Autodesk Inventor part; units mm, degrees
(part 2 of 18)
  ellipse E96 centre (-10059.4953, -10011.6684) end of major axis (-10059.5216, -10011.169) minor radius 0.0016 (-10059.5115, -10011.3383) -> (-10059.5141, -10011.3335) ccw
  line L123 (-10061.6074, -10010.6749) -> (-10061.6853, -10010.6709)
  line L124 (-10061.783, -10009.7539) -> (-10061.5792, -10009.7642)
  line L125 (-10061.6156, -10010.9399) -> (-10061.5672, -10009.3749)
  ellipse E97 centre (-10061.4209, -10009.295) end of major axis (-10061.3805, -10008.496) minor radius 0.143 (-10061.3805, -10008.496) -> (-10061.5409, -10009.0123) ccw
  line L126 (-10061.571, -10010.9422) -> (-10061.6156, -10010.9399)
  ellipse E98 centre (-10059.4556, -10009.3943) end of major axis (-10059.4152, -10008.5953) minor radius 0.143 (-10059.3426, -10008.7344) -> (-10059.5711, -10009.0745) ccw
  line L127 (-10059.4152, -10008.5953) -> (-10061.3805, -10008.496)
  line L128 (-10061.571, -10009.4991) -> (-10061.8166, -10009.4867)
  line L129 (-10061.6156, -10010.9399) -> (-10061.8118, -10010.93)
  line L130 (-10063.3919, -10010.8501) -> (-10063.6427, -10010.8374)
  ellipse E99 centre (-10075.0796, -10008.6044) end of major axis (-10074.9741, -10006.5171) minor radius 0.3735 (-10074.9741, -10006.5171) -> (-10075.403, -10007.9525) ccw
  ellipse E100 centre (-10074.1952, -10008.6491) end of major axis (-10074.0897, -10006.5618) minor radius 0.3735 (-10073.8946, -10006.9512) -> (-10074.5173, -10007.9854) ccw
  line L131 (-10074.9741, -10006.5171) -> (-10074.0897, -10006.5618)
  ellipse E101 centre (-10074.1952, -10008.6491) end of major axis (-10074.1195, -10007.151) minor radius 0.2681 (-10074.0146, -10007.2936) -> (-10074.4107, -10009.8693) ccw
  ellipse E102 centre (-10059.4556, -10009.3943) end of major axis (-10059.4303, -10008.895) minor radius 0.0894 (-10059.3634, -10009.2087) -> (-10059.5442, -10009.3788) ccw
  line L132 (-10059.8989, -10015.0944) -> (-10059.8016, -10014.6093)
  line L133 (-10059.8016, -10014.6093) -> (-10059.814, -10014.6001)
  ellipse E103 centre (-10059.3774, -10016.4493) end of major axis (-10059.1723, -10015.676) minor radius 0.1421 (-10059.1558, -10016.0937) -> (-10059.1723, -10015.676) ccw
  line L134 (-10059.1723, -10015.676) -> (-10059.8752, -10015.4896)
  line L135 (-10062.35, -10019.5456) -> (-10062.8067, -10019.5173)
  line L136 (-10060.3914, -10027.4914) -> (-10060.3323, -10027.2827)
  ellipse E104 centre (-10060.3058, -10027.7257) end of major axis (-10060.5274, -10028.4943) minor radius 0.1461 (-10060.3074, -10027.284) -> (-10060.3936, -10027.516) ccw
  ellipse E105 centre (-10059.3611, -10027.9981) end of major axis (-10059.2226, -10027.5176) minor radius 0.0913 (-10059.2273, -10027.8389) -> (-10059.4494, -10027.9748) ccw
  ellipse E106 centre (-10059.3611, -10027.9981) end of major axis (-10059.1395, -10027.2294) minor radius 0.1461 (-10059.1442, -10027.7299) -> (-10059.4076, -10027.6709) ccw
  line L137 (-10059.1395, -10027.2294) -> (-10059.5247, -10027.1183)
  ellipse E107 centre (-10061.1947, -10025.0322) end of major axis (-10061.4841, -10025.778) minor radius 0.0025 (-10061.4641, -10025.7239) -> (-10061.4841, -10025.778) ccw
  ellipse E108 centre (-10061.1947, -10025.0322) end of major axis (-10060.9052, -10024.2864) minor radius 0.0025 (-10061.4579, -10025.7077) -> (-10061.4588, -10025.71) ccw
  line L138 (-10060.6601, -10023.6469) -> (-10060.6559, -10023.6361)
  line L139 (-10060.6559, -10023.6361) -> (-10059.7237, -10023.9979)
  ellipse E109 centre (-10059.3301, -10025.7558) end of major axis (-10059.0407, -10025.01) minor radius 0.0025 (-10059.215, -10025.4653) -> (-10059.2158, -10025.4549) ccw
  line L140 (-10061.4747, -10025.7816) -> (-10061.4841, -10025.778)
  line L141 (-10059.0407, -10025.01) -> (-10059.9651, -10024.6512)
  line L142 (-10060.6559, -10023.6361) -> (-10060.6965, -10023.6203)
  line L143 (-10060.8833, -10023.5478) -> (-10065.815, -10021.6339)
  ellipse E110 centre (-10059.9849, -10023.8481) end of major axis (-10060.3776, -10022.9558) minor radius 0.1687 (-10059.9009, -10023.6263) -> (-10060.3456, -10022.9572) ccw
  line L144 (-10060.3456, -10022.9572) -> (-10064.6064, -10021.3037)
  line L145 (-10059.9009, -10023.6263) -> (-10059.7237, -10023.9979)
  line L146 (-10059.7237, -10023.9979) -> (-10059.9563, -10024.6128)
  line L147 (-10059.948, -10024.5763) -> (-10059.7237, -10023.9979)
  ellipse E111 centre (-10059.3301, -10025.7558) end of major axis (-10059.1492, -10025.2896) minor radius 0.0015 (-10059.2152, -10025.4628) -> (-10059.2156, -10025.4573) ccw
  line L148 (-10061.1673, -10013.709) -> (-10061.4116, -10012.4308)
  ellipse E112 centre (-10061.4191, -10012.3797) end of major axis (-10061.5691, -10011.5939) minor radius 0.0022 (-10061.4497, -10012.231) -> (-10061.4116, -10012.4308) ccw
  ellipse E113 centre (-10061.4191, -10012.3797) end of major axis (-10061.5691, -10011.5939) minor radius 0.0022 (-10061.5691, -10011.5939) -> (-10061.4792, -10012.076) ccw
  line L149 (-10061.5626, -10011.5927) -> (-10061.5691, -10011.5939)
  line L150 (-10061.4353, -10010.9692) -> (-10061.5403, -10010.0292)
  ellipse E114 centre (-10074.1883, -10011.2004) end of major axis (-10074.3345, -10009.7075) minor radius 0.2416 (-10074.3956, -10009.773) -> (-10074.4256, -10009.8711) ccw
  ellipse E115 centre (-10074.1883, -10011.2004) end of major axis (-10074.392, -10009.1204) minor radius 0.3366 (-10074.4689, -10009.1938) -> (-10074.4718, -10009.1998) ccw
  ellipse E116 centre (-10059.4546, -10009.7574) end of major axis (-10059.4058, -10010.255) minor radius 0.0805 (-10059.453, -10010.1908) -> (-10059.4275, -10010.2411) ccw
  ellipse E117 centre (-10059.4546, -10009.7574) end of major axis (-10059.5033, -10009.2598) minor radius 0.0805 (-10059.5175, -10009.2701) -> (-10059.5437, -10009.3842) ccw
  ellipse E118 centre (-10061.3909, -10025.8081) end of major axis (-10061.2388, -10025.0226) minor radius 0.0868 (-10061.4894, -10025.8618) -> (-10061.5648, -10026.4557) ccw
  line L151 (-10061.4894, -10025.8618) -> (-10061.4567, -10025.6836)
  line L152 (-10061.2304, -10013.1017) -> (-10061.302, -10012.8602)
  ellipse E119 centre (-10061.3135, -10012.8141) end of major axis (-10061.5409, -10012.0472) minor radius 0.0022 (-10061.3592, -10012.6675) -> (-10061.302, -10012.8602) ccw
  ellipse E120 centre (-10061.3135, -10012.8141) end of major axis (-10061.5409, -10012.0472) minor radius 0.0022 (-10061.3802, -10012.5962) -> (-10061.3795, -10012.5988) ccw
  ellipse E121 centre (-10061.3135, -10012.8141) end of major axis (-10061.5409, -10012.0472) minor radius 0.0022 (-10061.5409, -10012.0477) -> (-10061.4673, -10012.3011) ccw
  line L153 (-10059.8961, -10014.0829) -> (-10060.2291, -10014.1817)
  line L154 (-10067.4297, -10016.1096) -> (-10067.4268, -10016.1197)
  line L155 (-10064.2229, -10015.3662) -> (-10067.0815, -10016.2141)
  line L156 (-10059.8993, -10014.0717) -> (-10059.8961, -10014.0829)
  line L157 (-10059.8961, -10014.0829) -> (-10059.936, -10014.1466)
  line L158 (-10059.8961, -10014.0829) -> (-10059.9646, -10013.8519)
  line L159 (-10061.4597, -10010.5107) -> (-10061.4635, -10010.4932)
  ellipse E122 centre (-10061.3479, -10010.4186) end of major axis (-10061.5106, -10009.6353) minor radius 0.1285 (-10061.5089, -10010.2574) -> (-10061.4635, -10010.4932) ccw
  line L160 (-10060.3618, -10010.9128) -> (-10060.3756, -10010.8496)
  ellipse E123 centre (-10059.4151, -10010.0173) end of major axis (-10059.3135, -10010.5069) minor radius 0.0803 (-10059.4497, -10010.2168) -> (-10059.2869, -10010.3723) ccw
  ellipse E124 centre (-10061.4428, -10028.7052) end of major axis (-10061.4376, -10029.5052) minor radius 0.1258 (-10061.5687, -10028.685) -> (-10061.4376, -10029.5052) ccw
  line L161 (-10061.5687, -10028.685) -> (-10061.5705, -10027.9704)
  line L162 (-10061.5725, -10027.1323) -> (-10061.5726, -10027.1107)
  line L163 (-10061.5726, -10027.1107) -> (-10061.5433, -10027.1105)
  ellipse E125 centre (-10059.4677, -10028.6922) end of major axis (-10059.4625, -10029.4922) minor radius 0.1258 (-10059.5871, -10028.4073) -> (-10059.5936, -10028.672) ccw
  line L164 (-10061.5726, -10027.1107) -> (-10062.1103, -10027.1142)
  line L165 (-10063.1147, -10027.1209) -> (-10063.6302, -10027.1243)
  ellipse E126 centre (-10075.1696, -10028.7957) end of major axis (-10075.1558, -10030.8856) minor radius 0.3286 (-10075.4962, -10028.958) -> (-10075.432, -10029.9867) ccw
  ellipse E127 centre (-10074.2808, -10028.7898) end of major axis (-10074.267, -10030.8798) minor radius 0.3286 (-10074.6056, -10029.0344) -> (-10074.5441, -10029.973) ccw
  ellipse E128 centre (-10074.2808, -10028.7898) end of major axis (-10074.2709, -10030.2898) minor radius 0.2359 (-10074.5075, -10028.3133) -> (-10074.258, -10030.2874) ccw
  ellipse E129 centre (-10059.4677, -10028.6922) end of major axis (-10059.4645, -10029.1922) minor radius 0.0786 (-10059.5435, -10028.8078) -> (-10059.4024, -10028.9872) ccw
  ellipse E130 centre (-10061.4829, -10026.279) end of major axis (-10061.5501, -10027.0761) minor radius 0.0022 (-10061.4921, -10026.3627) -> (-10061.5501, -10027.0761) ccw
  line L166 (-10061.5412, -10027.0769) -> (-10061.5501, -10027.0761)
  line L167 (-10061.1675, -10013.708) -> (-10064.1267, -10014.2572)
  line L168 (-10061.0399, -10013.9291) -> (-10061.1256, -10013.7034)
  line L169 (-10061.0399, -10013.9291) -> (-10061.3186, -10012.3815)
  ellipse E131 centre (-10061.4026, -10012.3529) end of major axis (-10061.5486, -10011.5664) minor radius 0.0775 (-10061.3186, -10012.3815) -> (-10061.5655, -10011.726) ccw
  ellipse E132 centre (-10061.4026, -10012.3529) end of major axis (-10061.2567, -10013.1395) minor radius 0.0775 (-10061.5654, -10011.7276) -> (-10061.5651, -10011.7329) ccw
  line L170 (-10061.5651, -10011.7329) -> (-10061.5627, -10011.7772)
  line L171 (-10061.006, -10013.9229) -> (-10061.0399, -10013.9291)
  line L172 (-10061.5148, -10011.5601) -> (-10061.5486, -10011.5664)
  line L173 (-10061.0399, -10013.9291) -> (-10062.4396, -10014.1889)
  line L174 (-10061.5324, -10011.3464) -> (-10062.0925, -10011.4011)
  line L175 (-10061.413, -10010.968) -> (-10061.51, -10010.0167)
  ellipse E133 centre (-10061.4701, -10009.9537) end of major axis (-10061.5479, -10009.1575) minor radius 0.046 (-10061.5593, -10009.2154) -> (-10061.51, -10010.0167) ccw
  line L176 (-10061.5682, -10011.6005) -> (-10062.0791, -10011.6504)
  ellipse E134 centre (-10075.2814, -10011.3029) end of major axis (-10075.4846, -10009.2228) minor radius 0.1201 (-10075.4962, -10009.236) -> (-10075.5025, -10009.9969) ccw
  ellipse E135 centre (-10074.3871, -10011.2156) end of major axis (-10074.5903, -10009.1355) minor radius 0.1201 (-10074.6056, -10009.1595) -> (-10074.6228, -10009.4041) ccw
  ellipse E136 centre (-10074.3871, -10011.2156) end of major axis (-10074.533, -10009.7227) minor radius 0.0862 (-10074.479, -10009.8773) -> (-10074.556, -10009.8863) ccw
  ellipse E137 centre (-10059.4829, -10009.7596) end of major axis (-10059.5315, -10009.2619) minor radius 0.0287 (-10059.5388, -10009.3031) -> (-10059.5392, -10009.3196) ccw
  line L177 (-10062.0933, -10026.8089) -> (-10061.5337, -10026.8636)
  ellipse E138 centre (-10061.4701, -10028.2403) end of major axis (-10061.5479, -10029.0365) minor radius 0.046 (-10061.5147, -10028.2236) -> (-10061.5593, -10028.9786) ccw
  line L178 (-10061.5147, -10028.2236) -> (-10061.4163, -10027.2258)
  ellipse E139 centre (-10075.2814, -10026.8911) end of major axis (-10075.4846, -10028.9712) minor radius 0.1201 (-10075.5025, -10028.1971) -> (-10075.4962, -10028.958) ccw
  ellipse E140 centre (-10074.3871, -10026.9784) end of major axis (-10074.5903, -10029.0585) minor radius 0.1201 (-10074.6228, -10028.7899) -> (-10074.6056, -10029.0344) ccw
  ellipse E141 centre (-10074.3871, -10026.9784) end of major axis (-10074.533, -10028.4713) minor radius 0.0862 (-10074.556, -10028.3077) -> (-10074.479, -10028.3167) ccw
  ellipse E142 centre (-10059.4829, -10028.4344) end of major axis (-10059.4343, -10027.9368) minor radius 0.0287 (-10059.4284, -10027.9558) -> (-10059.4497, -10027.9771) ccw
  ellipse E143 centre (-10059.4829, -10028.4344) end of major axis (-10059.5315, -10028.9321) minor radius 0.0287 (-10059.534, -10028.7144) -> (-10059.5203, -10028.9087) ccw
  line L179 (-10064.1321, -10023.9836) -> (-10061.1995, -10024.5278)
  ellipse E144 centre (-10061.4026, -10025.8411) end of major axis (-10061.5486, -10026.6276) minor radius 0.0775 (-10061.5648, -10026.4557) -> (-10061.3382, -10025.9171) ccw
  line L180 (-10061.3382, -10025.9171) -> (-10061.0521, -10024.4386)
  line L181 (-10061.5148, -10026.6339) -> (-10061.5486, -10026.6276)
  line L182 (-10061.3493, -10013.5219) -> (-10061.4817, -10011.9546)
  ellipse E145 centre (-10061.4829, -10011.915) end of major axis (-10061.5501, -10011.1179) minor radius 0.0022 (-10061.492, -10011.8329) -> (-10061.4817, -10011.9546) ccw
  ellipse E146 centre (-10061.4829, -10011.915) end of major axis (-10061.5501, -10011.1179) minor radius 0.0022 (-10061.5501, -10011.1179) -> (-10061.492, -10011.8327) ccw
  line L183 (-10061.2053, -10013.5098) -> (-10061.3493, -10013.5219)
  line L184 (-10061.5412, -10011.1171) -> (-10061.5501, -10011.1179)
  line L185 (-10061.3493, -10013.5219) -> (-10063.059, -10013.6661)
  line L186 (-10064.1551, -10013.7586) -> (-10064.1846, -10013.7611)
  line L187 (-10061.7547, -10009.9957) -> (-10061.5864, -10009.9968)
  line L188 (-10061.558, -10011.1248) -> (-10061.5686, -10009.5555)
  ellipse E147 centre (-10061.4428, -10009.4888) end of major axis (-10061.4376, -10008.6888) minor radius 0.1258 (-10061.5458, -10009.0552) -> (-10061.5686, -10009.5555) ccw
  line L189 (-10061.5498, -10011.1249) -> (-10061.558, -10011.1248)
  line L190 (-10061.558, -10011.1248) -> (-10062.1079, -10011.1212)
  line L191 (-10063.1128, -10011.1146) -> (-10063.9018, -10011.1094)
  ellipse E148 centre (-10075.1696, -10009.3983) end of major axis (-10075.1834, -10011.4883) minor radius 0.3286 (-10075.432, -10008.2073) -> (-10075.4962, -10009.236) ccw
  ellipse E149 centre (-10074.2808, -10009.4042) end of major axis (-10074.2946, -10011.4941) minor radius 0.3286 (-10074.5441, -10008.2209) -> (-10074.6056, -10009.1595) ccw
  ellipse E150 centre (-10074.2808, -10009.4042) end of major axis (-10074.2709, -10007.9042) minor radius 0.2359 (-10074.2349, -10007.9221) -> (-10074.5075, -10009.8807) ccw
  ellipse E151 centre (-10060.4553, -10009.4953) end of major axis (-10060.4606, -10010.2952) minor radius 0.1258 (-10060.5811, -10009.562) -> (-10060.5678, -10009.8834) ccw
  ellipse E152 centre (-10059.4677, -10009.5018) end of major axis (-10059.4645, -10009.0018) minor radius 0.0786 (-10059.5212, -10009.1492) -> (-10059.5435, -10009.3862) ccw
  line L192 (-10060.3705, -10027.2925) -> (-10060.3681, -10027.2809)
  ellipse E153 centre (-10059.4151, -10028.1767) end of major axis (-10059.3135, -10027.6871) minor radius 0.0803 (-10059.2869, -10027.8217) -> (-10059.4497, -10027.9772) ccw
  ellipse E154 centre (-10061.3135, -10025.3799) end of major axis (-10061.5409, -10026.1468) minor radius 0.0022 (-10061.4677, -10025.8942) -> (-10061.5409, -10026.1463) ccw
  line L193 (-10065.4273, -10022.5831) -> (-10067.279, -10022.0339)
  line L194 (-10067.4279, -10022.0746) -> (-10067.4306, -10022.084)
  ellipse E155 centre (-10063.9396, -10011.2006) end of major axis (-10064.1437, -10010.36) minor radius 0.1481 (-10064.0618, -10011.3216) -> (-10064.0429, -10011.3917) ccw
  ellipse E156 centre (-10063.9396, -10011.2006) end of major axis (-10064.1437, -10010.36) minor radius 0.1481 (-10064.1077, -10011.131) -> (-10064.0971, -10011.178) ccw
  ellipse E157 centre (-10064.7515, -10028.8711) end of major axis (-10064.763, -10028.4142) minor radius 0.0765 (-10064.8032, -10028.491) -> (-10064.8181, -10029.044) ccw
  ellipse E158 centre (-10064.7515, -10028.8711) end of major axis (-10064.7297, -10029.7358) minor radius 0.1448 (-10064.8817, -10028.3695) -> (-10064.6507, -10029.578) ccw
  ellipse E159 centre (-10065.737, -10028.8959) end of major axis (-10065.7152, -10029.7606) minor radius 0.1448 (-10065.8826, -10028.6784) -> (-10065.7152, -10029.7606) ccw
  line L195 (-10065.7152, -10029.7606) -> (-10064.7297, -10029.7358)
  ellipse E160 centre (-10064.0118, -10026.1549) end of major axis (-10064.0736, -10027.0177) minor radius 0.0025 (-10064.0074, -10026.0573) -> (-10064.0564, -10026.8016) ccw
  line L196 (-10064.4832, -10026.9884) -> (-10064.0736, -10027.0177)
  ellipse E161 centre (-10063.7189, -10010.2205) end of major axis (-10063.6288, -10011.0808) minor radius 0.037 (-10063.8048, -10009.3643) -> (-10063.6232, -10011.0615) ccw
  ellipse E162 centre (-10064.7126, -10010.3246) end of major axis (-10064.8027, -10009.4643) minor radius 0.037 (-10064.8027, -10009.4643) -> (-10064.7062, -10010.7042) ccw
  line L197 (-10064.8027, -10009.4643) -> (-10063.809, -10009.3602)
  line L198 (-10064.4873, -10011.1707) -> (-10063.6288, -10011.0808)
  ellipse E163 centre (-10063.7189, -10027.9735) end of major axis (-10063.809, -10028.8338) minor radius 0.037 (-10063.6288, -10027.1132) -> (-10063.8048, -10028.8297) ccw
  ellipse E164 centre (-10064.7126, -10027.8694) end of major axis (-10064.8027, -10028.7297) minor radius 0.037 (-10064.7062, -10027.4898) -> (-10064.8027, -10028.7297) ccw
  line L199 (-10064.4873, -10027.0233) -> (-10063.6288, -10027.1132)
  line L200 (-10064.8027, -10028.7297) -> (-10063.809, -10028.8338)
  ellipse E165 centre (-10064.0118, -10012.0391) end of major axis (-10064.0736, -10011.1763) minor radius 0.0025 (-10064.0564, -10011.3924) -> (-10064.0074, -10012.1367) ccw
  line L201 (-10064.4832, -10011.2056) -> (-10064.0736, -10011.1763)
  ellipse E166 centre (-10064.7515, -10009.3229) end of major axis (-10064.7399, -10008.866) minor radius 0.0765 (-10064.8181, -10009.1499) -> (-10064.8032, -10009.703) ccw
  ellipse E167 centre (-10064.7515, -10009.3229) end of major axis (-10064.7297, -10008.4582) minor radius 0.1448 (-10064.6507, -10008.616) -> (-10064.8817, -10009.8245) ccw
  ellipse E168 centre (-10065.737, -10009.2981) end of major axis (-10065.7152, -10008.4333) minor radius 0.1448 (-10065.7152, -10008.4333) -> (-10065.8826, -10009.5156) ccw
  line L202 (-10065.7152, -10008.4333) -> (-10064.7297, -10008.4582)
  ellipse E169 centre (-10061.9748, -10012.6358) end of major axis (-10061.8761, -10013.082) minor radius 0.0015 (-10062.0482, -10012.3082) -> (-10061.8783, -10013.0704) ccw
  ellipse E170 centre (-10061.9748, -10012.6358) end of major axis (-10062.1616, -10011.7912) minor radius 0.0028 (-10062.0681, -10012.2252) -> (-10061.826, -10013.3162) ccw
  ellipse E171 centre (-10062.9512, -10012.8518) end of major axis (-10063.138, -10012.0072) minor radius 0.0028 (-10063.1133, -10012.1253) -> (-10062.8248, -10013.4322) ccw
  line L203 (-10062.9607, -10009.3224) -> (-10062.8582, -10009.3108)
  line L204 (-10062.9607, -10028.8715) -> (-10062.8582, -10028.8832)
  ellipse E172 centre (-10061.9748, -10025.5582) end of major axis (-10061.8761, -10025.1119) minor radius 0.0015 (-10061.8783, -10025.1236) -> (-10062.0482, -10025.8858) ccw
  ellipse E173 centre (-10061.9748, -10025.5582) end of major axis (-10061.788, -10024.7136) minor radius 0.0028 (-10061.8594, -10025.0267) -> (-10062.0681, -10025.9688) ccw
  ellipse E174 centre (-10062.9512, -10025.3422) end of major axis (-10062.7644, -10024.4976) minor radius 0.0028 (-10062.8655, -10024.9437) -> (-10063.1133, -10026.0687) ccw
  ellipse E175 centre (-10061.849, -10012.6268) end of major axis (-10061.9493, -10012.1809) minor radius 0.0774 (-10061.8216, -10012.4274) -> (-10061.7949, -10013.03) ccw
  ellipse E176 centre (-10061.849, -10012.6268) end of major axis (-10062.0389, -10011.7829) minor radius 0.1465 (-10061.8751, -10013.0848) -> (-10061.8447, -10013.1717) ccw
  ellipse E177 centre (-10061.849, -10012.6268) end of major axis (-10062.0389, -10011.7829) minor radius 0.1465 (-10061.8216, -10012.1727) -> (-10062.0708, -10011.8238) ccw
  line L205 (-10062.0718, -10011.7903) -> (-10062.0389, -10011.7829)
  ellipse E178 centre (-10061.849, -10025.5672) end of major axis (-10061.9493, -10026.013) minor radius 0.0774 (-10061.7916, -10025.1585) -> (-10061.7969, -10025.68) ccw
  ellipse E179 centre (-10061.849, -10025.5672) end of major axis (-10061.6591, -10024.7233) minor radius 0.1465 (-10061.8678, -10025.0874) -> (-10061.8751, -10025.1092) ccw
  ellipse E180 centre (-10061.849, -10025.5672) end of major axis (-10062.0389, -10026.4111) minor radius 0.1465 (-10062.0708, -10026.3701) -> (-10061.7584, -10025.8106) ccw
  line L206 (-10062.0718, -10026.4037) -> (-10062.0389, -10026.4111)
  ellipse E181 centre (-10062.9958, -10013.8608) end of major axis (-10063.3087, -10013.0544) minor radius 0.0027 (-10063.066, -10013.687) -> (-10062.9308, -10014.0352) ccw
  ellipse E182 centre (-10063.928, -10014.2226) end of major axis (-10064.241, -10013.4162) minor radius 0.0027 (-10064.0503, -10013.9142) -> (-10063.9315, -10014.2209) ccw
  ellipse E183 centre (-10063.1313, -10011.2831) end of major axis (-10063.371, -10010.4519) minor radius 0.158 (-10063.3308, -10011.1485) -> (-10063.276, -10011.3513) ccw
  ellipse E184 centre (-10063.1313, -10011.2831) end of major axis (-10063.371, -10010.4519) minor radius 0.158 (-10063.4048, -10010.7574) -> (-10063.3436, -10011.0949) ccw
  ellipse E185 centre (-10062.9557, -10028.9766) end of major axis (-10062.9327, -10029.433) minor radius 0.0817 (-10063.0378, -10028.7491) -> (-10062.8805, -10028.8806) ccw
  ellipse E186 centre (-10062.9557, -10028.9766) end of major axis (-10062.9121, -10029.8405) minor radius 0.1546 (-10063.1086, -10028.5065) -> (-10062.8058, -10028.8928) ccw
  ellipse E187 centre (-10063.9384, -10029.0263) end of major axis (-10063.8947, -10029.8902) minor radius 0.1546 (-10064.0988, -10028.8034) -> (-10063.8947, -10029.8902) ccw
  line L207 (-10063.8947, -10029.8902) -> (-10062.9121, -10029.8405)
  ellipse E188 centre (-10062.0737, -10026.3901) end of major axis (-10062.0977, -10026.8465) minor radius 0.0015 (-10062.0523, -10025.9956) -> (-10062.0605, -10026.1623) ccw
  ellipse E189 centre (-10062.0737, -10026.3901) end of major axis (-10062.1191, -10027.2539) minor radius 0.0028 (-10062.0495, -10025.8857) -> (-10062.0717, -10026.4037) ccw
  ellipse E190 centre (-10063.0724, -10026.3376) end of major axis (-10063.027, -10025.4738) minor radius 0.0028 (-10063.0348, -10025.5948) -> (-10063.0434, -10025.7481) ccw
  ellipse E191 centre (-10063.0724, -10026.3376) end of major axis (-10063.1178, -10027.2014) minor radius 0.0028 (-10063.0482, -10025.8356) -> (-10063.1178, -10027.2014) ccw
  line L208 (-10063.1178, -10027.2014) -> (-10062.1191, -10027.2539)
  ellipse E192 centre (-10063.2676, -10012.8641) end of major axis (-10063.0883, -10013.7103) minor radius 0.1305 (-10063.0883, -10013.7103) -> (-10063.447, -10012.0179) ccw
  ellipse E193 centre (-10064.2347, -10013.0691) end of major axis (-10064.0553, -10013.9153) minor radius 0.1305 (-10064.1494, -10013.8029) -> (-10064.3594, -10012.2648) ccw
  line L209 (-10064.3655, -10012.2126) -> (-10063.447, -10012.0179)
  line L210 (-10064.0553, -10013.9153) -> (-10063.0883, -10013.7103)
  ellipse E194 centre (-10061.7665, -10010.0544) end of major axis (-10061.8177, -10009.6003) minor radius 0.0097
  ellipse E195 centre (-10061.7665, -10010.0544) end of major axis (-10061.6696, -10010.914) minor radius 0.0184 (-10061.6841, -10010.671) -> (-10061.6679, -10010.8984) ccw
  ellipse E196 centre (-10062.76, -10010.1665) end of major axis (-10062.6631, -10011.026) minor radius 0.0184 (-10062.8569, -10009.3069) -> (-10062.6761, -10010.9693) ccw
  line L211 (-10062.8569, -10009.3069) -> (-10061.8635, -10009.1949)
  line L212 (-10062.1172, -10010.9644) -> (-10061.6696, -10010.914)
  ellipse E197 centre (-10061.7665, -10028.1396) end of major axis (-10061.8177, -10028.5937) minor radius 0.0097
  ellipse E198 centre (-10061.7665, -10028.1396) end of major axis (-10061.8635, -10028.9991) minor radius 0.0184 (-10061.6717, -10027.2834) -> (-10061.6865, -10027.5497) ccw
  ellipse E199 centre (-10062.76, -10028.0275) end of major axis (-10062.8569, -10028.8871) minor radius 0.0184 (-10062.6761, -10027.2246) -> (-10062.8569, -10028.8871) ccw
  line L213 (-10062.8569, -10028.8871) -> (-10061.8635, -10028.9991)
  ellipse E200 centre (-10063.2676, -10025.3299) end of major axis (-10063.447, -10026.1761) minor radius 0.1305 (-10063.447, -10026.1761) -> (-10063.0883, -10024.4837) ccw
  ellipse E201 centre (-10064.2347, -10025.1249) end of major axis (-10064.414, -10025.9711) minor radius 0.1305 (-10064.3594, -10025.9292) -> (-10064.1022, -10024.3099) ccw
  line L214 (-10064.0553, -10024.2787) -> (-10063.0883, -10024.4837)
  line L215 (-10064.3655, -10025.9814) -> (-10063.447, -10026.1761)
  ellipse E202 centre (-10062.0737, -10011.8039) end of major axis (-10062.0498, -10012.2602) minor radius 0.0015 (-10062.0605, -10012.0317) -> (-10062.0523, -10012.1984) ccw
  ellipse E203 centre (-10062.0737, -10011.8039) end of major axis (-10062.1191, -10010.9401) minor radius 0.0028 (-10062.0717, -10011.7903) -> (-10062.0495, -10012.3083) ccw
  ellipse E204 centre (-10063.0724, -10011.8564) end of major axis (-10063.1178, -10010.9925) minor radius 0.0028 (-10063.0434, -10012.4459) -> (-10063.0348, -10012.5992) ccw
  ellipse E205 centre (-10063.0724, -10011.8564) end of major axis (-10063.1178, -10010.9925) minor radius 0.0028 (-10063.1178, -10010.9925) -> (-10063.0482, -10012.3584) ccw
  line L216 (-10063.1178, -10010.9925) -> (-10062.1191, -10010.9401)
  ellipse E206 centre (-10062.9557, -10009.2174) end of major axis (-10062.9327, -10008.7609) minor radius 0.0817 (-10062.8805, -10009.3133) -> (-10063.0378, -10009.4448) ccw
  ellipse E207 centre (-10062.9557, -10009.2174) end of major axis (-10062.9121, -10008.3535) minor radius 0.1546 (-10062.8058, -10009.3011) -> (-10063.1086, -10009.6875) ccw
  ellipse E208 centre (-10063.9384, -10009.1677) end of major axis (-10063.8947, -10008.3038) minor radius 0.1546 (-10063.8947, -10008.3038) -> (-10064.0988, -10009.3906) ccw
  line L217 (-10063.8947, -10008.3038) -> (-10062.9121, -10008.3535)
  ellipse E209 centre (-10063.1313, -10026.9109) end of major axis (-10062.8917, -10026.0798) minor radius 0.158 (-10063.276, -10026.8426) -> (-10063.2973, -10026.9171) ccw
  ellipse E210 centre (-10062.9958, -10024.3332) end of major axis (-10062.6828, -10023.5268) minor radius 0.0027 (-10062.9482, -10024.2033) -> (-10063, -10024.3367) ccw
  ellipse E211 centre (-10063.928, -10023.9714) end of major axis (-10063.6151, -10023.165) minor radius 0.0027 (-10063.9488, -10024.0176) -> (-10064.0218, -10024.206) ccw
  ellipse E212 centre (-10067.6052, -10010.5425) end of major axis (-10067.6885, -10009.6815) minor radius 0.2215 (-10067.8219, -10009.9617) -> (-10067.8329, -10010.0578) ccw
  ellipse E213 centre (-10067.6052, -10027.6515) end of major axis (-10067.522, -10026.7905) minor radius 0.2215 (-10067.8329, -10028.1362) -> (-10067.8219, -10028.2322) ccw
  ellipse E214 centre (-10066.5988, -10028.7392) end of major axis (-10066.6018, -10028.2822) minor radius 0.0719 (-10066.6682, -10028.6016) -> (-10066.6627, -10028.9319) ccw
  ellipse E215 centre (-10066.5988, -10028.7392) end of major axis (-10066.5931, -10029.6042) minor radius 0.136 (-10066.7338, -10028.5952) -> (-10066.6007, -10029.6029) ccw
  ellipse E216 centre (-10067.5863, -10028.7457) end of major axis (-10067.5806, -10029.6107) minor radius 0.136 (-10067.6888, -10028.1502) -> (-10067.5953, -10029.6057) ccw
  ellipse E217 centre (-10065.688, -10010.3657) end of major axis (-10065.7324, -10009.9109) minor radius 0.0263 (-10065.7294, -10009.9132) -> (-10065.735, -10009.9138) ccw
  ellipse E218 centre (-10065.688, -10010.3657) end of major axis (-10065.7721, -10009.5048) minor radius 0.0497 (-10065.7634, -10009.5146) -> (-10065.7188, -10010.5507) ccw
  ellipse E219 centre (-10066.6816, -10010.4628) end of major axis (-10066.7657, -10009.6019) minor radius 0.0497 (-10066.7657, -10009.6019) -> (-10066.7379, -10010.3963) ccw
  line L218 (-10066.7657, -10009.6019) -> (-10065.7721, -10009.5048)
  ellipse E220 centre (-10065.688, -10027.8282) end of major axis (-10065.7324, -10028.2831) minor radius 0.0263 (-10065.735, -10028.2802) -> (-10065.7294, -10028.2807) ccw
  ellipse E221 centre (-10065.688, -10027.8282) end of major axis (-10065.7721, -10028.6891) minor radius 0.0497 (-10065.7188, -10027.6433) -> (-10065.7634, -10028.6794) ccw
  ellipse E222 centre (-10066.6816, -10027.7312) end of major axis (-10066.7657, -10028.5921) minor radius 0.0497 (-10066.7379, -10027.7977) -> (-10066.7657, -10028.5921) ccw
  line L219 (-10066.7657, -10028.5921) -> (-10065.7721, -10028.6891)
  ellipse E223 centre (-10066.5988, -10009.4548) end of major axis (-10066.5957, -10008.9978) minor radius 0.0719 (-10066.6627, -10009.2621) -> (-10066.6682, -10009.5924) ccw
  ellipse E224 centre (-10066.5988, -10009.4548) end of major axis (-10066.5931, -10008.5898) minor radius 0.136 (-10066.6007, -10008.5911) -> (-10066.7338, -10009.5988) ccw
  ellipse E225 centre (-10067.5863, -10009.4483) end of major axis (-10067.5806, -10008.5833) minor radius 0.136 (-10067.5953, -10008.5882) -> (-10067.6888, -10010.0437) ccw
  ellipse E226 centre (-10139.4756, -10019.097) end of major axis (-10140.2159, -10019.0311) minor radius 0.1949 (-10139.6973, -10018.892) -> (-10139.2539, -10019.302) ccw
  line L220 (-10137.2443, -10019.302) -> (-10139.2539, -10019.302)
  line L221 (-10137.687, -10018.892) -> (-10139.6973, -10018.892)
  ellipse E227 centre (-10139.476, -10016.9627) end of major axis (-10140.2301, -10016.8195) minor radius 0.1955 (-10139.6765, -10016.7356) -> (-10140.0057, -10017.0105) ccw
  line L222 (-10117.7101, -10019.4461) -> (-10118.5143, -10019.3619)
  line L223 (-10138.1344, -10016.8969) -> (-10139.6765, -10016.7356)
  ellipse E228 centre (-10139.476, -10021.2313) end of major axis (-10140.2434, -10021.2474) minor radius 0.1955 (-10140.2268, -10021.2055) -> (-10139.2331, -10021.412) ccw
  line L224 (-10138.2283, -10021.3069) -> (-10139.2331, -10021.412)
  line L225 (-10117.7101, -10018.7479) -> (-10118.5143, -10018.8321)
  ellipse E229 centre (-10137.4656, -10019.097) end of major axis (-10138.2026, -10019.0308) minor radius 0.1948 (-10137.687, -10018.892) -> (-10137.2443, -10019.302) ccw
  line L226 (-10120.709, -10019.302) -> (-10137.2443, -10019.302)
  line L227 (-10120.709, -10018.892) -> (-10137.687, -10018.892)
  ellipse E230 centre (-10137.4655, -10016.9315) end of major axis (-10138.2178, -10016.7793) minor radius 0.1955 (-10137.6632, -10016.702) -> (-10137.9302, -10017.0006) ccw
  line L228 (-10110.6961, -10020.2656) -> (-10117.7103, -10019.446)
  line L229 (-10119.0212, -10018.8801) -> (-10137.6632, -10016.702)
  line L230 (-10110.6942, -10019.302) -> (-10117.1987, -10019.302)
  line L231 (-10110.6942, -10018.892) -> (-10117.1987, -10018.892)
  ellipse E231 centre (-10137.4655, -10021.2625) end of major axis (-10138.2327, -10021.2878) minor radius 0.1955 (-10138.1925, -10021.2224) -> (-10137.2204, -10021.4402) ccw
  line L232 (-10119.0212, -10019.3139) -> (-10137.2204, -10021.4402)
  line L233 (-10110.6961, -10017.9284) -> (-10117.7103, -10018.7479)
  ellipse E232 centre (-10141.5037, -10019.097) end of major axis (-10142.2686, -10019.0331) minor radius 0.1955 (-10141.7266, -10018.892) -> (-10141.2808, -10019.302) ccw
  line L234 (-10141.2598, -10019.302) -> (-10141.2808, -10019.302)
  line L235 (-10141.7036, -10018.892) -> (-10141.7266, -10018.892)
  ellipse E233 centre (-10141.4817, -10019.097) end of major axis (-10142.2246, -10019.0313) minor radius 0.1949 (-10141.7036, -10018.892) -> (-10141.2598, -10019.302) ccw
  line L236 (-10139.2539, -10019.302) -> (-10141.2598, -10019.302)
  line L237 (-10139.6973, -10018.892) -> (-10141.7036, -10018.892)
  ellipse E234 centre (-10141.4825, -10016.9789) end of major axis (-10142.238, -10016.8432) minor radius 0.1955 (-10141.6851, -10016.7538) -> (-10141.2799, -10017.2041) ccw
  ellipse E235 centre (-10110.6856, -10019.8981) end of major axis (-10110.6663, -10019.694) minor radius 0 (-10110.6663, -10019.694) -> (-10110.6896, -10019.9398) ccw
  line L238 (-10118.5134, -10019.362) -> (-10119.0213, -10019.3139)
  line L239 (-10123.4722, -10018.892) -> (-10141.2799, -10017.2041)
  line L240 (-10110.6663, -10019.694) -> (-10114.8017, -10019.302)
  line L241 (-10140.196, -10016.895) -> (-10141.6851, -10016.7538)
  ellipse E236 centre (-10141.4825, -10021.215) end of major axis (-10142.25, -10021.2236) minor radius 0.1955 (-10141.7237, -10021.032) -> (-10141.2413, -10021.3981) ccw
  ellipse E237 centre (-10110.6856, -10018.2959) end of major axis (-10110.6663, -10018.5) minor radius 0 (-10110.6896, -10018.2541) -> (-10110.6663, -10018.5) ccw
  line L242 (-10110.6663, -10018.5) -> (-10114.8017, -10018.892)
  line L243 (-10140.2126, -10021.3006) -> (-10141.2413, -10021.3981)
  line L244 (-10118.5134, -10018.832) -> (-10119.0213, -10018.8801)
  line L245 (-10123.4722, -10019.302) -> (-10141.7237, -10021.032)
  line L246 (-10067.9499, -10028.149) -> (-10067.9649, -10028.1233)
  line L247 (-10068.0699, -10028.2074) -> (-10068.0683, -10028.2003)
  line L248 (-10068.0546, -10028.2338) -> (-10068.0699, -10028.2074)
  line L249 (-10068.0699, -10028.2074) -> (-10068.0998, -10028.2043)
  line L250 (-10068.1024, -10029.8123) -> (-10068.1016, -10029.795)
  line L251 (-10068.1016, -10029.795) -> (-10068.1215, -10029.7476)
  line L252 (-10068.1648, -10029.6441) -> (-10068.1786, -10029.611)
  line L253 (-10068.2503, -10029.4398) -> (-10068.2604, -10029.4157)
  line L254 (-10068.2694, -10029.6089) -> (-10068.2604, -10029.4157)
  line L255 (-10068.2352, -10029.6906) -> (-10068.2694, -10029.6089)
  line L256 (-10068.2604, -10029.4157) -> (-10068.2616, -10029.4157)
  line L257 (-10068.2694, -10029.6089) -> (-10068.3259, -10029.6103)
  line L258 (-10070.1697, -10029.6568) -> (-10070.1701, -10029.6568)
  line L259 (-10072.2637, -10029.7096) -> (-10072.2885, -10029.7102)
  line L260 (-10068.3213, -10029.0451) -> (-10068.3058, -10029.0822)
  line L261 (-10068.3344, -10029.0455) -> (-10068.3213, -10029.0451)
  line L262 (-10068.3213, -10029.0451) -> (-10068.3158, -10028.9277)
  line L263 (-10068.3088, -10028.7778) -> (-10068.2862, -10028.2936)
  line L264 (-10068.2389, -10009.8616) -> (-10068.2412, -10009.8347)
  line L265 (-10068.2616, -10009.5912) -> (-10068.2624, -10009.5825)
  line L266 (-10068.3257, -10009.3274) -> (-10068.3185, -10009.302)
  line L267 (-10068.3207, -10009.3866) -> (-10068.3257, -10009.3274)
  line L268 (-10068.3257, -10009.3274) -> (-10068.3443, -10009.3269)
  line L269 (-10068.3685, -10008.9068) -> (-10068.275, -10008.9091)
  line L270 (-10068.2898, -10008.7329) -> (-10068.275, -10008.9091)
  line L271 (-10072.3104, -10008.6316) -> (-10072.2921, -10008.6321)
  line L272 (-10070.1905, -10008.685) -> (-10070.1693, -10008.6856)
  line L273 (-10068.357, -10008.7312) -> (-10068.2898, -10008.7329)
  line L274 (-10068.275, -10008.9091) -> (-10068.2399, -10008.7853)
  line L275 (-10068.1599, -10008.5028) -> (-10068.1563, -10008.4898)
  line L276 (-10068.2898, -10008.7329) -> (-10068.2449, -10008.5744)
  line L277 (-10068.0699, -10008.4244) -> (-10068.0752, -10008.4429)
  line L278 (-10068.2161, -10009.9662) -> (-10068.2138, -10009.9534)
  line L279 (-10067.9958, -10029.7471) -> (-10068.0035, -10029.9726)
  line L280 (-10067.965, -10030.0606) -> (-10068.0035, -10029.9726)
  line L281 (-10067.9544, -10029.745) -> (-10067.965, -10030.0606)
  line L282 (-10067.965, -10030.0606) -> (-10068.0119, -10030.063)
  line L283 (-10068.0569, -10030.2704) -> (-10068.0505, -10030.0799)
  line L284 (-10068.1118, -10030.2731) -> (-10068.0569, -10030.2704)
  line L285 (-10068.0505, -10030.0799) -> (-10068.2279, -10029.6737)
  line L286 (-10068.2344, -10029.8641) -> (-10068.2279, -10029.6737)
  line L287 (-10068.0569, -10030.2704) -> (-10068.2344, -10029.8641)
  line L288 (-10068.2279, -10029.6737) -> (-10068.2343, -10029.674)
  line L289 (-10068.2344, -10029.8641) -> (-10068.2438, -10029.8645)
  line L290 (-10072.3033, -10029.4965) -> (-10072.2729, -10029.4949)
  line L291 (-10068.2516, -10009.1768) -> (-10068.2518, -10009.1737)
  line L292 (-10068.2642, -10008.9583) -> (-10068.2676, -10008.8995)
  line L293 (-10068.3051, -10009.0066) -> (-10068.2676, -10008.8995)
  line L294 (-10068.3019, -10009.0624) -> (-10068.3051, -10009.0066)
  line L295 (-10068.2676, -10008.8995) -> (-10068.2722, -10008.8993)
  line L296 (-10068.3051, -10009.0066) -> (-10068.3629, -10009.0037)
  line L297 (-10070.1883, -10008.9114) -> (-10070.2002, -10008.9108)
  line L298 (-10068.2431, -10008.5982) -> (-10068.2391, -10008.5984)
  line L299 (-10068.2495, -10008.4181) -> (-10068.2391, -10008.5984)
  line L300 (-10068.2686, -10008.4171) -> (-10068.2495, -10008.4181)
  line L301 (-10068.2391, -10008.5984) -> (-10068.0656, -10008.1036)
  line L302 (-10068.076, -10007.9233) -> (-10068.0656, -10008.1036)
  line L303 (-10068.2495, -10008.4181) -> (-10068.076, -10007.9233)
  line L304 (-10068.076, -10007.9233) -> (-10068.1288, -10007.9206)
  line L305 (-10067.9779, -10008.0732) -> (-10068.0154, -10008.1803)
  line L306 (-10068.0269, -10008.0708) -> (-10067.9779, -10008.0732)
  line L307 (-10068.0154, -10008.1803) -> (-10068.0001, -10008.4467)
  line L308 (-10067.9779, -10008.0732) -> (-10067.9563, -10008.4489)
  line L309 (-10068.2662, -10029.2321) -> (-10068.2878, -10029.1652)
  line L310 (-10068.3013, -10029.3533) -> (-10068.2878, -10029.1652)
  line L311 (-10068.2665, -10029.461) -> (-10068.3013, -10029.3533)
  line L312 (-10068.2878, -10029.1652) -> (-10068.3384, -10029.1655)
  line L313 (-10070.191, -10029.1777) -> (-10070.6135, -10029.1805)
  line L314 (-10068.3013, -10029.3533) -> (-10068.3448, -10029.3536)
  line L315 (-10070.1998, -10029.3658) -> (-10070.2058, -10029.3658)
  line L316 (-10072.3032, -10029.3797) -> (-10072.3299, -10029.3798)
  line L317 (-10068.246, -10010.0982) -> (-10068.3065, -10009.3732)
  line L318 (-10068.3359, -10009.4774) -> (-10068.3065, -10009.3732)
  line L319 (-10068.3128, -10009.7535) -> (-10068.3359, -10009.4774)
  line L320 (-10068.3065, -10009.3732) -> (-10068.3164, -10009.3732)
  line L321 (-10068.3359, -10009.4774) -> (-10068.3581, -10009.4773)
  line L322 (-10072.3335, -10009.4511) -> (-10072.3645, -10009.4509)
  line L323 (-10086.4602, -10026.53) -> (-10086.5642, -10027.5252)
  line L324 (-10087.3594, -10030.3237) -> (-10087.0615, -10027.4732)
  ellipse E238 centre (-10087.134, -10028.1706) end of major axis (-10087.3941, -10030.657) minor radius 0.0002 (-10087.3594, -10030.3237) -> (-10087.3941, -10030.657) ccw
  line L325 (-10085.5062, -10030.8545) -> (-10087.3941, -10030.657)
  line L326 (-10086.5642, -10010.6688) -> (-10086.4602, -10011.664)
  line L327 (-10087.0615, -10010.7208) -> (-10087.3594, -10007.8703)
  ellipse E239 centre (-10087.134, -10010.0234) end of major axis (-10087.3941, -10007.537) minor radius 0.0002 (-10087.3941, -10007.537) -> (-10087.3594, -10007.8703) ccw
  line L328 (-10087.3941, -10007.537) -> (-10085.5062, -10007.3394)
  ellipse E240 centre (-10082.6437, -10027.8966) end of major axis (-10082.6727, -10028.1449) minor radius 0
  ellipse E241 centre (-10082.5188, -10026.8281) end of major axis (-10082.5881, -10027.421) minor radius 0 (-10082.5822, -10027.3702) -> (-10082.5822, -10027.3702) ccw
  ellipse E242 centre (-10082.9263, -10030.3171) end of major axis (-10082.8339, -10029.5267) minor radius 0 (-10082.9672, -10030.6666) -> (-10082.9671, -10030.6667) ccw
  line L329 (-10082.5824, -10027.3701) -> (-10083.0307, -10031.2103)
  ellipse E243 centre (-10082.7794, -10029.06) end of major axis (-10083.0695, -10031.5431) minor radius 0.0001 (-10083.0298, -10031.2029) -> (-10083.0695, -10031.543) ccw
  line L330 (-10085.5138, -10030.9202) -> (-10085.1815, -10028.0738)
  ellipse E244 centre (-10085.2625, -10028.7699) end of major axis (-10085.5526, -10031.253) minor radius 0.0001 (-10085.5138, -10030.9202) -> (-10085.5526, -10031.253) ccw
  line L331 (-10083.0695, -10031.5431) -> (-10085.5526, -10031.253)
  ellipse E245 centre (-10082.118, -10023.3981) end of major axis (-10083.1044, -10031.8407) minor radius 0.0004 (-10083.055, -10031.4191) -> (-10082.967, -10030.6669) ccw
  line L332 (-10084.5689, -10027.1382) -> (-10084.6849, -10028.1318)
  ellipse E246 centre (-10082.6437, -10010.2974) end of major axis (-10082.6147, -10010.5457) minor radius 0
  ellipse E247 centre (-10082.5188, -10011.3658) end of major axis (-10082.5881, -10010.773) minor radius 0 (-10082.5822, -10010.8238) -> (-10082.5822, -10010.8238) ccw
  ellipse E248 centre (-10082.118, -10014.7958) end of major axis (-10083.1044, -10006.3533) minor radius 0.0004 (-10082.967, -10007.5271) -> (-10083.055, -10006.7749) ccw
  ellipse E249 centre (-10082.7794, -10009.134) end of major axis (-10083.0695, -10006.6509) minor radius 0.0001 (-10083.055, -10006.7749) -> (-10083.0307, -10006.9837) ccw
  line L333 (-10083.0307, -10006.9837) -> (-10082.5824, -10010.8238)
  line L334 (-10085.1815, -10010.1202) -> (-10085.5138, -10007.2738)
  ellipse E250 centre (-10085.2625, -10009.4241) end of major axis (-10085.5526, -10006.941) minor radius 0.0001 (-10085.5526, -10006.941) -> (-10085.5138, -10007.2738) ccw
  line L335 (-10085.5526, -10006.941) -> (-10083.0695, -10006.6509)
  ellipse E251 centre (-10082.9263, -10007.8768) end of major axis (-10082.8339, -10008.6673) minor radius 0 (-10082.9671, -10007.5272) -> (-10082.9672, -10007.5274) ccw
  line L336 (-10084.6849, -10010.0622) -> (-10084.5689, -10011.0558)
  line L337 (-10088.3757, -10026.0301) -> (-10088.4701, -10027.0259)
  line L338 (-10089.2382, -10029.8315) -> (-10088.9678, -10026.9787)
  ellipse E252 centre (-10089.0339, -10027.6762) end of major axis (-10089.2698, -10030.165) minor radius 0 (-10089.2382, -10029.8315) -> (-10089.2698, -10030.165) ccw
  line L339 (-10087.3617, -10030.3459) -> (-10089.2698, -10030.165)
  line L340 (-10088.5565, -10015.0089) -> (-10088.5709, -10015.097)
  line L341 (-10088.5709, -10023.097) -> (-10088.5565, -10023.1851)
  line L342 (-10088.7771, -10024.8816) -> (-10088.9053, -10024.097)
  line L343 (-10088.9053, -10014.097) -> (-10088.7771, -10013.3124)
  line L344 (-10088.4701, -10011.1681) -> (-10088.3757, -10012.1639)
  line L345 (-10088.9678, -10011.2153) -> (-10089.2382, -10008.3625)
  ellipse E253 centre (-10089.0339, -10010.5178) end of major axis (-10089.2698, -10008.0289) minor radius 0 (-10089.2698, -10008.0289) -> (-10089.2382, -10008.3624) ccw
  line L346 (-10089.2698, -10008.0289) -> (-10087.3617, -10007.8481)
  spline S0 degree 3 poles (-10089.3554, -10025.373) (-10089.3752, -10025.3281) (-10089.4144, -10025.2393) (-10089.4706, -10025.1064) (-10089.5241, -10024.9757) (-10089.591, -10024.8053) (-10089.6686, -10024.5967) (-10089.7237, -10024.4292) (-10089.7508, -10024.3468) knots 0 0 0 0 0.13379 0.264806 0.393183 0.519054 0.763783 1 1 1 1
  line L347 (-10088.8289, -10025.4281) -> (-10089.3554, -10025.373)
  spline S1 degree 3 poles (-10089.7131, -10026.5008) (-10089.712, -10026.5142) (-10089.7098, -10026.5406) (-10089.7078, -10026.5798) (-10089.7066, -10026.6176) (-10089.7065, -10026.6539) (-10089.7075, -10026.6885) (-10089.7097, -10026.7213) (-10089.7129, -10026.7522) (-10089.7171, -10026.7811) (-10089.7222, -10026.808) (-10089.7283, -10026.8328) (-10089.7352, -10026.8556) (-10089.7429, -10026.8763) (-10089.7515, -10026.895) (-10089.761, -10026.9119) (-10089.7715, -10026.9274) (-10089.7795, -10026.9365) (-10089.7834, -10026.941) knots 0 0 0 0 0.088475 0.174424 0.25743 0.337089 0.413015 0.484966 0.552919 0.616878 0.676853 0.732867 0.784956 0.833184 0.87778 0.920162 0.960829 1 1 1 1
  ellipse E254 centre (-10089.0274, -10022.2409) end of major axis (-10089.5956, -10027.6723) minor radius 0.0004 (-10089.3554, -10025.373) -> (-10089.5956, -10027.6723) ccw
  line L348 (-10089.85, -10027.3585) -> (-10089.5956, -10027.6723)
  line L349 (-10089.0391, -10027.7305) -> (-10089.5956, -10027.6723)
  spline S2 degree 3 poles (-10089.4919, -10022.2469) (-10089.5162, -10022.2043) (-10089.5642, -10022.12) (-10089.6335, -10021.9938) (-10089.6999, -10021.8693) (-10089.7837, -10021.7069) (-10089.8821, -10021.5074) (-10089.9539, -10021.3465) (-10089.9892, -10021.2675) knots 0 0 0 0 0.133763 0.26476 0.393126 0.518994 0.763738 1 1 1 1
  line L350 (-10089.3102, -10022.2469) -> (-10089.4919, -10022.2469)
  line L351 (-10089.4919, -10015.9471) -> (-10089.3102, -10015.9471)
  spline S3 degree 3 poles (-10089.9892, -10016.9265) (-10089.9539, -10016.8475) (-10089.8821, -10016.6865) (-10089.7837, -10016.4871) (-10089.6999, -10016.3247) (-10089.6335, -10016.2002) (-10089.5642, -10016.0739) (-10089.5162, -10015.9897) (-10089.4919, -10015.9471) knots 0 0 0 0 0.236262 0.481006 0.606874 0.73524 0.866237 1 1 1 1
  line L352 (-10089.9892, -10021.2675) -> (-10089.9892, -10016.9265)
  ellipse E255 centre (-10089.525, -10019.097) end of major axis (-10089.525, -10024.058) minor radius 0.5163 (-10089.9598, -10016.4224) -> (-10089.9892, -10016.9265) ccw
  ellipse E256 centre (-10089.525, -10019.097) end of major axis (-10089.525, -10024.058) minor radius 0.5163 (-10089.9892, -10021.2675) -> (-10089.9598, -10021.7716) ccw
  ellipse E257 centre (-10089.0277, -10019.097) end of major axis (-10089.0277, -10013.636) minor radius 0.5683 (-10089.1658, -10013.7997) -> (-10089.4919, -10015.9471) ccw
  ellipse E258 centre (-10089.0277, -10019.097) end of major axis (-10089.0277, -10024.558) minor radius 0.5683 (-10089.4919, -10022.2469) -> (-10089.1658, -10024.3943) ccw
  line L353 (-10089.3554, -10012.821) -> (-10088.8289, -10012.7659)
  spline S4 degree 3 poles (-10089.7508, -10013.8471) (-10089.7237, -10013.7648) (-10089.6686, -10013.5973) (-10089.591, -10013.3886) (-10089.5241, -10013.2183) (-10089.4706, -10013.0875) (-10089.4144, -10012.9547) (-10089.3752, -10012.8659) (-10089.3554, -10012.821) knots 0 0 0 0 0.236217 0.480946 0.606817 0.735194 0.86621 1 1 1 1
  spline S5 degree 3 poles (-10089.7836, -10011.2534) (-10089.7796, -10011.2581) (-10089.7714, -10011.2677) (-10089.7607, -10011.2839) (-10089.7508, -10011.3018) (-10089.7419, -10011.3215) (-10089.734, -10011.343) (-10089.727, -10011.3663) (-10089.7211, -10011.3912) (-10089.7161, -10011.4179) (-10089.7122, -10011.4463) (-10089.7094, -10011.4765) (-10089.7075, -10011.5084) (-10089.7067, -10011.5422) (-10089.7068, -10011.5777) (-10089.708, -10011.6149) (-10089.7101, -10011.6538) (-10089.7122, -10011.6802) (-10089.7133, -10011.6936) knots 0 0 0 0 0.040391 0.082789 0.1275 0.174786 0.22486 0.277901 0.334055 0.393442 0.45616 0.522411 0.592561 0.666584 0.744418 0.825989 0.911213 1 1 1 1
  ellipse E259 centre (-10089.0274, -10015.9531) end of major axis (-10089.5956, -10010.5217) minor radius 0.0004 (-10089.5956, -10010.5217) -> (-10089.3554, -10012.821) ccw
  line L354 (-10089.85, -10010.8355) -> (-10089.5956, -10010.5217)
  line L355 (-10089.0391, -10010.4635) -> (-10089.5956, -10010.5217)
  spline S6 degree 3 poles (-10091.2821, -10024.901) (-10091.3023, -10024.8563) (-10091.3424, -10024.7678) (-10091.3999, -10024.6355) (-10091.4546, -10024.5053) (-10091.5232, -10024.3356) (-10091.6029, -10024.1278) (-10091.6596, -10023.9608) (-10091.6874, -10023.8787) knots 0 0 0 0 0.13379 0.264806 0.393183 0.519054 0.763783 1 1 1 1
  line L356 (-10089.4849, -10025.0713) -> (-10091.2821, -10024.901)
  line L357 (-10091.6874, -10023.8787) -> (-10091.612, -10023.083)
  ellipse E260 centre (-10091.4826, -10021.7182) end of major axis (-10091.9507, -10026.6571) minor radius 0.0001 (-10091.9347, -10026.4873) -> (-10091.9507, -10026.6571) ccw
  ellipse E261 centre (-10091.4826, -10021.7182) end of major axis (-10091.9507, -10026.6571) minor radius 0.0001 (-10091.6874, -10023.8787) -> (-10091.814, -10025.2141) ccw
  spline S7 degree 3 poles (-10091.814, -10025.2141) (-10091.7982, -10025.2657) (-10091.7671, -10025.3667) (-10091.7263, -10025.5161) (-10091.6912, -10025.6591) (-10091.6628, -10025.7949) (-10091.6409, -10025.9237) (-10091.6264, -10026.0453) (-10091.6207, -10026.1419) (-10091.6211, -10026.2135) (-10091.6238, -10026.2617) (-10091.6289, -10026.3058) (-10091.6361, -10026.3455) (-10091.6453, -10026.3809) (-10091.6594, -10026.4203) (-10091.6822, -10026.4617) (-10091.7201, -10026.4988) (-10091.7675, -10026.5198) (-10091.821, -10026.5224) (-10091.878, -10026.5112) (-10091.9152, -10026.4955) (-10091.9347, -10026.4873) knots 0 0 0 0 0.104135 0.203976 0.298889 0.388275 0.471711 0.551067 0.624597 0.658204 0.689291 0.717816 0.743784 0.767218 0.788166 0.824633 0.857384 0.888881 0.922221 0.959245 1 1 1 1
  ellipse E262 centre (-10090.9848, -10021.7654) end of major axis (-10091.5002, -10027.2021) minor radius 0.0001 (-10091.2821, -10024.901) -> (-10091.5002, -10027.2021) ccw
  line L358 (-10091.9507, -10026.6571) -> (-10091.5002, -10027.2021)
  ellipse E263 centre (-10091.8085, -10025.1562) end of major axis (-10091.6659, -10023.6517) minor radius 0 (-10091.9347, -10026.4878) -> (-10091.8218, -10025.2969) ccw
  line L359 (-10089.85, -10027.3585) -> (-10091.5002, -10027.2021)
  spline S8 degree 3 poles (-10091.4056, -10022.2469) (-10091.4299, -10022.2043) (-10091.4779, -10022.12) (-10091.5473, -10021.9938) (-10091.6138, -10021.8693) (-10091.6977, -10021.7069) (-10091.7962, -10021.5074) (-10091.8681, -10021.3465) (-10091.9034, -10021.2675) knots 0 0 0 0 0.133768 0.264768 0.393136 0.519004 0.763746 1 1 1 1
  line L360 (-10089.6915, -10022.2469) -> (-10091.4056, -10022.2469)
  line L361 (-10091.4056, -10015.9471) -> (-10089.6915, -10015.9471)
  spline S9 degree 3 poles (-10091.9034, -10016.9265) (-10091.8681, -10016.8475) (-10091.7962, -10016.6865) (-10091.6977, -10016.4871) (-10091.6138, -10016.3247) (-10091.5473, -10016.2002) (-10091.4779, -10016.0739) (-10091.4299, -10015.9897) (-10091.4056, -10015.9471) knots 0 0 0 0 0.236254 0.480996 0.606864 0.735232 0.866232 1 1 1 1
  line L362 (-10091.9034, -10021.2675) -> (-10091.9034, -10016.9265)